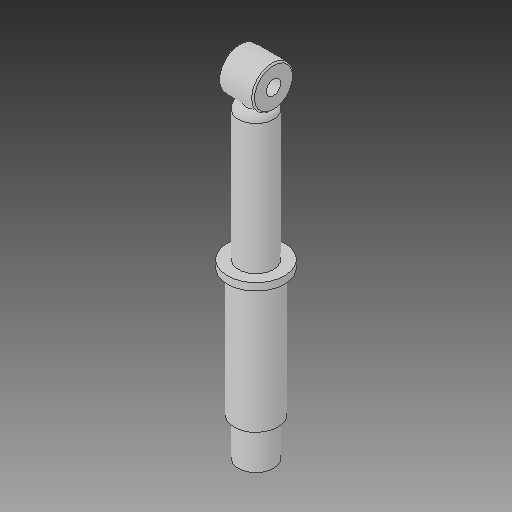
# Autodesk Inventor part: スプリングその１
Saved by Autodesk Inventor 2018 (Build 220112000, 112)
## iProperties
Created: 2017-09-09
Part Number: スプリングその１
Material: 一般
Document SubType Name: Modeling
Designer: Kenta
Density: 1 g/cm^3
Appearance: 既定
Mass: 128.525 g
Surface Area: 267.877 cm^2
Volume: 128.525 cm^3
Author: Kenta
Autodesk Inventor part; units mm, degrees
ref_plane "YZ Plane" through (0, 0, 0) normal (1, 0, 0) x (0, 1, 0)
ref_plane "XZ Plane" through (0, 0, 0) normal (0, 1, 0) x (-1, 0, 0)
ref_plane "XY Plane" through (0, 0, 0) normal (0, 0, 1) x (1, 0, 0)
sketch "スケッチ1" plane through (0, 0, 0) normal (0, 1, 0) x (-1, 0, 0)
  circle A0 centre (0, 0) radius 12
  dimension "d0" = 24
  constraints: 1 centre point, 1 coincident
  measures "d0" diameter of A0
extrude "押し出し1" add sketch "スケッチ1" along normal blind 94
sketch "スケッチ3" plane through (0, 0, 0) normal (1, 0, 0) x (0, 1, 0)
  circle A0 centre (108.1, 0) radius 14
  line L0 (94, -12) -> (94, 12) projected
  point P0 (0, 0)
  dimension "d3" = 28
  dimension "d4" = 14.1
  constraints: 1 centre point
  measures "d3" diameter of A0
  measures "d4" distance from line of L0 A0.centre
extrude "押し出し2" add sketch "スケッチ3" along normal mid plane 24
sketch "スケッチ4" plane through (12, 108.1, 0) normal (1, 0, 0) x (0, 0, -1)
  point P0 (0, -108.1)
  point P1 (0, 0)
hole "穴1" at (12, 108.1, 0) direction (-1, 0, 0) diameter 10 end through all
fillet "フィレット2" radius 5 1 edges at (12, 94, 0)
fillet "フィレット3" radius 1 1 edges at (12, 94.1, 0)
fillet "フィレット4" radius 1 1 edges at (-12, 94.1, 0)
sketch "スケッチ5" plane through (0, 0, 0) normal (0, -1, 0) x (1, 0, 0)
  circle A0 centre (0, 0) radius 19.5
  dimension "d18" = 39
  constraints: 1 centre point, 1 coincident
  measures "d18" diameter of A0
extrude "押し出し3" add sketch "スケッチ5" along normal blind 5
sketch "スケッチ6" plane through (0, -5, 0) normal (0, -1, 0) x (1, 0, 0)
  circle A0 centre (0, 0) radius 15
  dimension "d21" = 30
  constraints: 1 centre point, 1 coincident
  measures "d21" diameter of A0
extrude "押し出し4" add sketch "スケッチ6" along normal blind 87
sketch "スケッチ7" plane through (0, -92, 0) normal (0, -1, 0) x (1, 0, 0)
  circle A0 centre (0, 0) radius 12
  dimension "d24" = 24
  constraints: 1 centre point, 1 coincident
  measures "d24" diameter of A0
extrude "押し出し5" add sketch "スケッチ7" along normal blind 26
sketch "スケッチ8" plane through (0, -118, 0) normal (0, -1, 0) x (1, 0, 0)
  point P0 (0, 0)
  point P1 (0, 0)
  constraints: 1 coincident
hole "穴2" at (0, -118, 0) direction (0, 1, 0) diameter 8 depth 113 tip angle 118
